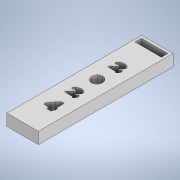
# Autodesk Inventor part: LegWithText2024
Saved by Autodesk Inventor 2021 (Build 250183000, 183)
## iProperties
Created: 2024-05-05
Part Number: LegWithText2024
Material: Generic
Document SubType Name: Modeling
Designer: brybr
Density: 1 g/cm^3
Appearance: Default
Author: brybr
Autodesk Inventor part; units mm, degrees
ref_plane "YZ Plane" through (0, 0, 0) normal (1, 0, 0) x (0, 1, 0)
ref_plane "XZ Plane" through (0, 0, 0) normal (0, 1, 0) x (-1, 0, 0)
ref_plane "XY Plane" through (0, 0, 0) normal (0, 0, 1) x (1, 0, 0)
sketch "Sketch1" plane through (0, 0, 0) normal (0, 0, 1) x (1, 0, 0)
  line L0 (-17.5, 6.5) -> (17.5, 6.5)
  line L1 (17.5, 6.5) -> (17.5, -6.5)
  line L2 (17.5, -6.5) -> (-17.5, -6.5)
  line L3 (-17.5, -6.5) -> (-17.5, 6.5)
  line L4 (-17.5, 6.5) -> (17.5, -6.5) construction
  line L5 (17.5, 6.5) -> (-17.5, -6.5) construction
  line L6 (-17.5, 6.5) -> (17.5, 6.5) construction
  point P0 (0, 0)
  dimension "d0" = 35
  dimension "d1" = 0
  dimension "d2" = 13
  constraints: 14 end point, 2 horizontal, 2 midpoint, 2 parallel, 1 collinear, 1 perpendicular
  measures "d0" distance of L0.start L0.end
  measures "d1" distance between parallel lines of L0 L6
  measures "d2" distance of L0.end L1.end
extrude "Extrusion1" add sketch "Sketch1" along normal blind 150
sketch "Sketch2" plane through (-17.5, 6.5, 0) normal (0, 1, 0) x (1, 0, 0)
  line L0 (2.8, -10.2) -> (32.2, -10.2)
  line L1 (32.2, -10.2) -> (32.2, -3)
  line L2 (32.2, -3) -> (2.8, -3)
  line L3 (2.8, -3) -> (2.8, -10.2)
  line L4 (2.8, -10.2) -> (32.2, -3) construction
  line L5 (32.2, -10.2) -> (2.8, -3) construction
  line L6 (2.8, -10.2) -> (32.2, -10.2) construction
  line L7 (2.8, -6.6) -> (0, -6.6)
  line L8 (0, 0) -> (0, -150) projected
  line L9 (35, 0) -> (35, -150) projected
  line L10 (35, -6.6) -> (32.2, -6.6)
  line L11 (35, 0) -> (0, 0) projected
  line L12 (2.8, -147) -> (32.2, -147)
  line L13 (32.2, -147) -> (32.2, -139.8)
  line L14 (32.2, -139.8) -> (2.8, -139.8)
  line L15 (2.8, -139.8) -> (2.8, -147)
  line L16 (2.8, -147) -> (32.2, -139.8) construction
  line L17 (32.2, -147) -> (2.8, -139.8) construction
  line L18 (2.8, -147) -> (32.2, -147) construction
  line L19 (2.8, -143.4) -> (0, -143.4)
  line L20 (35, -143.4) -> (32.2, -143.4)
  line L21 (35, -150) -> (0, -150) projected
  point P0 (17.5, 0)
  point P1 (17.5, -6.6)
  point P2 (17.5, -143.4)
  dimension "d6" = 29.4
  dimension "d7" = 0
  dimension "d8" = 7.2
  dimension "d9" = 3
  dimension "d12" = 29.4
  dimension "d13" = 0
  dimension "d14" = 7.2
  dimension "d15" = 3
  constraints: 36 end point, 8 midpoint, 6 horizontal, 6 point on line, 4 collinear, 4 parallel, 2 perpendicular
  measures "d6" distance of L0.start L0.end
  measures "d7" distance between parallel lines of L0 L6
  measures "d8" distance of L1.end L0.end
  measures "d9" distance between parallel lines of L11 L2
  measures "d12" distance of L12.start L12.end
  measures "d13" distance between parallel lines of L12 L18
  measures "d14" distance of L13.end L12.end
  measures "d15" distance between parallel lines of L21 L12
extrude "Extrusion2" cut sketch "Sketch2" against normal through all contours L3 L2 L1 L0
sketch "Sketch3" plane through (-17.5, 6.5, 0) normal (0, 1, 0) x (1, 0, 0)
  line L0 (6.4393, -10.6292) -> (29.3125, -10.6292) construction
  line L1 (29.3125, -10.6292) -> (29.3125, -150.0931) construction
  line L2 (29.3125, -150.0931) -> (6.4393, -150.0931) construction
  line L3 (6.4393, -150.0931) -> (6.4393, -10.6292) construction
  line L4 (19.7721, -49.3927) -> (12.7083, -49.3927)
  spline S0 degree 2 poles (12.7083, -49.3927) (11.5573, -49.3927) (11.5573, -48.6414) knots 0 0 0 1 1 1
  spline S1 degree 2 poles (11.5573, -48.6414) (11.5573, -48.3022) (12.0056, -47.7812) (13.096, -46.7513) knots 0 0 0 1 2 2 2
  spline S2 degree 2 poles (13.096, -46.7513) (15.071, -44.8975) (15.9918, -43.6011) knots 0 0 0 1 1 1
  spline S3 degree 2 poles (15.9918, -43.6011) (16.4886, -42.4985) (16.4886, -41.9532) knots 0 0 0 1 1 1
  spline S4 degree 2 poles (16.4886, -41.9532) (16.4886, -41.5292) (16.0161, -41.0445) (15.6041, -41.0445) knots 0 0 0 1 2 2 2
  spline S5 degree 2 poles (15.6041, -41.0445) (15.18, -41.0445) (14.756, -41.2626) (13.8957, -41.9896) knots 0 0 0 1 2 2 2
  spline S6 degree 2 poles (13.8957, -41.9896) (13.6291, -42.2077) (13.1808, -42.2077) knots 0 0 0 1 1 1
  spline S7 degree 2 poles (13.1808, -42.2077) (12.5993, -42.2077) (11.6542, -41.3353) (11.6542, -40.778) knots 0 0 0 1 2 2 2
  spline S8 degree 2 poles (11.6542, -40.778) (11.6542, -40.3175) (12.466, -39.2028) (13.0112, -38.7909) knots 0 0 0 1 2 2 2
  spline S9 degree 2 poles (13.0112, -38.7909) (15.3981, -37.0825) (18.197, -37.0825) knots 0 0 0 1 1 1
  spline S10 degree 2 poles (18.197, -37.0825) (20.3295, -37.0825) (21.735, -37.9185) knots 0 0 0 1 1 1
  spline S11 degree 2 poles (21.735, -37.9185) (22.3892, -38.3062) (23.201, -39.7117) (23.201, -40.475) knots 0 0 0 1 2 2 2
  spline S12 degree 2 poles (23.201, -40.475) (23.201, -42.3894) (20.2568, -44.6309) knots 0 0 0 1 1 1
  spline S13 degree 2 poles (20.2568, -44.6309) (19.7964, -45.261) (19.7964, -45.5276) knots 0 0 0 1 1 1
  spline S14 degree 2 poles (19.7964, -45.5276) (19.7964, -45.7214) (20.1962, -46.0122) (20.4991, -46.0122) knots 0 0 0 1 2 2 2
  spline S15 degree 2 poles (20.4991, -46.0122) (21.323, -46.0122) (21.9773, -45.37) knots 0 0 0 1 1 1
  spline S16 degree 2 poles (21.9773, -45.37) (22.3529, -45.0066) (22.6679, -44.8127) (22.9345, -44.8127) knots 0 0 0 1 2 2 2
  spline S17 degree 2 poles (22.9345, -44.8127) (24.0613, -44.8127) (24.0613, -46.5696) knots 0 0 0 1 1 1
  spline S18 degree 2 poles (24.0613, -46.5696) (24.0613, -47.3935) (23.4434, -49.0655) (22.6195, -49.744) knots 0 0 0 1 2 2 2
  spline S19 degree 2 poles (22.6195, -49.744) (22.3165, -50.362) (21.5653, -50.362) knots 0 0 0 1 1 1
  spline S20 degree 2 poles (21.5653, -50.362) (21.2382, -50.362) (20.8384, -50.0833) (20.7293, -49.8531) knots 0 0 0 1 2 2 2
  spline S21 degree 2 poles (20.7293, -49.8531) (20.4628, -49.5138) (20.1962, -49.3927) (19.7721, -49.3927) knots 0 0 0 1 2 2 2
  spline S22 degree 2 poles (17.7366, -61.1046) (19.2027, -61.1046) (20.5718, -61.8315) knots 0 0 0 1 1 1
  spline S23 degree 2 poles (20.5718, -61.8315) (22.4256, -62.8008) (23.3222, -64.7031) knots 0 0 0 1 1 1
  spline S24 degree 2 poles (23.3222, -64.7031) (24.0007, -66.0965) (24.0007, -67.6595) knots 0 0 0 1 1 1
  spline S25 degree 2 poles (24.0007, -67.6595) (24.0007, -70.531) (21.7955, -72.3727) knots 0 0 0 1 1 1
  spline S26 degree 2 poles (21.7955, -72.3727) (20.1114, -73.7661) (17.9547, -73.7661) knots 0 0 0 1 1 1
  spline S27 degree 2 poles (17.9547, -73.7661) (15.5678, -73.7661) (13.8836, -72.2031) knots 0 0 0 1 1 1
  spline S28 degree 2 poles (13.8836, -72.2031) (11.9086, -70.3735) (11.9086, -67.3081) knots 0 0 0 1 1 1
  spline S29 degree 2 poles (11.9086, -67.3081) (11.9086, -64.3396) (13.7261, -62.6312) knots 0 0 0 1 1 1
  spline S30 degree 2 poles (13.7261, -62.6312) (15.3254, -61.1046) (17.7366, -61.1046) knots 0 0 0 1 1 1
  spline S31 degree 2 poles (17.4821, -64.6183) (16.7552, -64.6183) (16.7552, -66.0359) knots 0 0 0 1 1 1
  spline S32 degree 2 poles (16.7552, -66.0359) (16.7552, -68.1441) (17.5427, -69.8041) knots 0 0 0 1 1 1
  spline S33 degree 2 poles (17.5427, -69.8041) (17.8093, -70.3493) (18.2091, -70.3493) knots 0 0 0 1 1 1
  spline S34 degree 2 poles (18.2091, -70.3493) (18.9361, -70.3493) (18.9361, -68.8832) knots 0 0 0 1 1 1
  spline S35 degree 2 poles (18.9361, -68.8832) (18.9361, -67.9745) (18.5484, -65.9026) (18.2455, -65.2604) knots 0 0 0 1 2 2 2
  spline S36 degree 2 poles (18.2455, -65.2604) (17.9547, -64.6425) (17.4821, -64.6183) knots 0 0 0 1 1 1
  line L5 (19.7721, -97.5822) -> (12.7083, -97.5822)
  spline S37 degree 2 poles (12.7083, -97.5822) (11.5573, -97.5822) (11.5573, -96.831) knots 0 0 0 1 1 1
  spline S38 degree 2 poles (11.5573, -96.831) (11.5573, -96.4917) (12.0056, -95.9707) (13.096, -94.9408) knots 0 0 0 1 2 2 2
  spline S39 degree 2 poles (13.096, -94.9408) (15.071, -93.087) (15.9918, -91.7906) knots 0 0 0 1 1 1
  spline S40 degree 2 poles (15.9918, -91.7906) (16.4886, -90.688) (16.4886, -90.1428) knots 0 0 0 1 1 1
  spline S41 degree 2 poles (16.4886, -90.1428) (16.4886, -89.7187) (16.0161, -89.2341) (15.6041, -89.2341) knots 0 0 0 1 2 2 2
  spline S42 degree 2 poles (15.6041, -89.2341) (15.18, -89.2341) (14.756, -89.4521) (13.8957, -90.1791) knots 0 0 0 1 2 2 2
  spline S43 degree 2 poles (13.8957, -90.1791) (13.6291, -90.3972) (13.1808, -90.3972) knots 0 0 0 1 1 1
  spline S44 degree 2 poles (13.1808, -90.3972) (12.5993, -90.3972) (11.6542, -89.5248) (11.6542, -88.9675) knots 0 0 0 1 2 2 2
  spline S45 degree 2 poles (11.6542, -88.9675) (11.6542, -88.5071) (12.466, -87.3924) (13.0112, -86.9804) knots 0 0 0 1 2 2 2
  spline S46 degree 2 poles (13.0112, -86.9804) (15.3981, -85.272) (18.197, -85.272) knots 0 0 0 1 1 1
  spline S47 degree 2 poles (18.197, -85.272) (20.3295, -85.272) (21.735, -86.108) knots 0 0 0 1 1 1
  spline S48 degree 2 poles (21.735, -86.108) (22.3892, -86.4958) (23.201, -87.9013) (23.201, -88.6646) knots 0 0 0 1 2 2 2
  spline S49 degree 2 poles (23.201, -88.6646) (23.201, -90.579) (20.2568, -92.8205) knots 0 0 0 1 1 1
  spline S50 degree 2 poles (20.2568, -92.8205) (19.7964, -93.4505) (19.7964, -93.7171) knots 0 0 0 1 1 1
  spline S51 degree 2 poles (19.7964, -93.7171) (19.7964, -93.911) (20.1962, -94.2017) (20.4991, -94.2017) knots 0 0 0 1 2 2 2
  spline S52 degree 2 poles (20.4991, -94.2017) (21.323, -94.2017) (21.9773, -93.5596) knots 0 0 0 1 1 1
  spline S53 degree 2 poles (21.9773, -93.5596) (22.3529, -93.1961) (22.6679, -93.0022) (22.9345, -93.0022) knots 0 0 0 1 2 2 2
  spline S54 degree 2 poles (22.9345, -93.0022) (24.0613, -93.0022) (24.0613, -94.7591) knots 0 0 0 1 1 1
  spline S55 degree 2 poles (24.0613, -94.7591) (24.0613, -95.583) (23.4434, -97.2551) (22.6195, -97.9336) knots 0 0 0 1 2 2 2
  spline S56 degree 2 poles (22.6195, -97.9336) (22.3165, -98.5515) (21.5653, -98.5515) knots 0 0 0 1 1 1
  spline S57 degree 2 poles (21.5653, -98.5515) (21.2382, -98.5515) (20.8384, -98.2728) (20.7293, -98.0426) knots 0 0 0 1 2 2 2
  spline S58 degree 2 poles (20.7293, -98.0426) (20.4628, -97.7034) (20.1962, -97.5822) (19.7721, -97.5822) knots 0 0 0 1 2 2 2
  line L6 (22.6437, -109.8999) -> (22.6437, -117.0607)
  spline S59 degree 2 poles (22.6437, -117.0607) (22.6437, -117.3151) (22.7164, -117.412) (22.8497, -117.412) knots 0 0 0 1 2 2 2
  line L7 (22.8497, -117.412) -> (23.4312, -117.412)
  spline S60 degree 2 poles (23.4312, -117.412) (23.9765, -117.3878) (24.0007, -118.2965) knots 0 0 0 1 1 1
  line L8 (24.0007, -118.2965) -> (24.0007, -120.3078)
  spline S61 degree 2 poles (24.0007, -120.3078) (24.0007, -121.0469) (23.2737, -121.1438) knots 0 0 0 1 1 1
  spline S62 degree 2 poles (23.2737, -121.1438) (22.9708, -121.1802) (22.8981, -121.2529) (22.8981, -121.5073) knots 0 0 0 1 2 2 2
  line L9 (22.8981, -121.5073) -> (22.8981, -122.7796)
  spline S63 degree 2 poles (22.8981, -122.7796) (22.9345, -123.5913) (22.0863, -123.6398) knots 0 0 0 1 1 1
  line L10 (22.0863, -123.6398) -> (18.5363, -123.6398)
  spline S64 degree 2 poles (18.5363, -123.6398) (18.0516, -123.6398) (17.7123, -123.2521) (17.7123, -122.7311) knots 0 0 0 1 2 2 2
  line L11 (17.7123, -122.7311) -> (17.7123, -121.6649)
  spline S65 degree 2 poles (17.7123, -121.6649) (17.7123, -121.3256) (17.5064, -121.1075) (17.1913, -121.1075) knots 0 0 0 1 2 2 2
  line L12 (17.1913, -121.1075) -> (13.1445, -121.1075)
  spline S66 degree 2 poles (13.1445, -121.1075) (12.3206, -121.1075) (11.6178, -120.3684) (11.6178, -119.5324) knots 0 0 0 1 2 2 2
  spline S67 degree 2 poles (11.6178, -119.5324) (11.6178, -118.5025) (11.848, -118.1632) knots 0 0 0 1 1 1
  spline S68 degree 2 poles (11.848, -118.1632) (12.1631, -117.1818) (13.9563, -115.4128) knots 0 0 0 1 1 1
  line L13 (13.9563, -115.4128) -> (16.1978, -112.3474)
  spline S69 degree 2 poles (16.1978, -112.3474) (18.197, -109.9605) (19.1663, -109.282) knots 0 0 0 1 1 1
  spline S70 degree 2 poles (19.1663, -109.282) (19.6146, -108.9791) (20.8989, -108.5792) (21.4563, -108.5792) knots 0 0 0 1 2 2 2
  spline S71 degree 2 poles (21.4563, -108.5792) (22.0742, -108.5792) (22.6437, -109.2335) (22.6437, -109.8999) knots 0 0 0 1 2 2 2
  line L14 (17.8577, -115.2796) -> (17.8577, -114.7707)
  spline S72 degree 2 poles (17.8577, -114.7707) (17.8577, -114.0558) (17.5548, -114.0558) knots 0 0 0 1 1 1
  spline S73 degree 2 poles (17.5548, -114.0558) (17.2762, -114.0558) (16.9975, -114.3951) knots 0 0 0 1 1 1
  line L15 (16.9975, -114.3951) -> (15.3981, -116.3579)
  spline S74 degree 2 poles (15.3981, -116.3579) (14.756, -117.1576) (14.756, -117.4484) knots 0 0 0 1 1 1
  spline S75 degree 2 poles (14.756, -117.4484) (14.756, -117.5695) (15.1437, -117.6665) (16.2705, -117.7028) knots 0 0 0 1 2 2 2
  line L16 (16.2705, -117.7028) -> (16.8642, -117.7149)
  spline S76 degree 2 poles (16.8642, -117.7149) (17.5427, -117.7149) (17.7729, -117.5695) (17.7972, -117.2909) knots 0 0 0 1 2 2 2
  spline S77 degree 2 poles (17.7972, -117.2909) (17.8577, -116.7335) (17.8577, -115.2796) knots 0 0 0 1 1 1
  point P0 (17.5, 0)
  constraints: 2 other
emboss "Emboss1" sketch "Sketch3" operation cut depth 20 direction (0, -1, 0)
sketch "Sketch4" plane through (-17.5, 6.5, 0) normal (0, 1, 0) x (1, 0, 0)
  line L0 (14.2568, -62.5548) -> (19.8156, -62.5548)
  line L1 (19.8156, -62.5548) -> (19.8156, -71.7543)
  line L2 (19.8156, -71.7543) -> (14.2568, -71.7543)
  line L3 (14.2568, -71.7543) -> (14.2568, -62.5548)
  arc A0 (14.2568, -117.6537) -> (17.5875, -113.3396) centre (16.3719, -115.8439) ccw
  line L4 (14.2568, -117.6537) -> (17.5875, -113.3396)
  point P0 (17.5, 0)
  constraints: 10 end point, 2 parallel, 2 point on circle, 1 centre point, 1 horizontal, 1 perpendicular
extrude "Extrusion3" cut sketch "Sketch4" against normal blind 13
body "Solid1"
